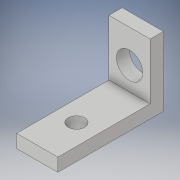
# Autodesk Inventor part: L形件
Saved by Autodesk Inventor 2017 (Build 210142000, 142)
## iProperties
Part Number: L形件
Material: 一般
Document SubType Name: Modeling
Designer: user
Density: 1 g/cm^3
Appearance: 預設
Author: user
Autodesk Inventor part; units mm, degrees
ref_plane "YZ Plane" through (0, 0, 0) normal (1, 0, 0) x (0, 1, 0)
ref_plane "XZ Plane" through (0, 0, 0) normal (0, 1, 0) x (-1, 0, 0)
ref_plane "XY Plane" through (0, 0, 0) normal (0, 0, 1) x (1, 0, 0)
sketch "草圖1" plane through (0, 0, 0) normal (1, 0, 0) x (0, 1, 0)
  line L0 (0, 0) -> (0, 32)
  line L1 (0, 32) -> (4, 32)
  line L2 (4, 32) -> (4, 4)
  line L3 (4, 4) -> (21, 4)
  line L4 (21, 4) -> (21, 0)
  line L5 (21, 0) -> (0, 0)
  dimension "d0" = 32
  dimension "d1" = 21
  dimension "d2" = 4
  dimension "d3" = 4
  constraints: 12 end point, 5 perpendicular, 1 vertical
  measures "d0" distance of L0.start L0.end
  measures "d1" distance of L4.end L0.start
  measures "d2" distance of L0.end L1.end
  measures "d3" distance between parallel lines of L5 L3
extrude "擠出1" add sketch "草圖1" along normal blind 12.5
sketch "草圖2" plane through (0, 4, 32) normal (0, 1, 0) x (1, 0, 0)
  circle A0 centre (6.25, 11.88) radius 2.5
  line L0 (0, 0) -> (12.5, 0) projected
  point P0 (0, 32)
  dimension "d6" = 5
  dimension "d7" = 11.88
  constraints: 1 centre point
  measures "d6" diameter of A0
  measures "d7" distance from line of A0.centre L0
extrude "擠出2" cut sketch "草圖2" against normal blind 12.5
sketch "草圖3" plane through (0, 4, 4) normal (0, 0, 1) x (1, 0, 0)
  circle A0 centre (6.25, 7) radius 4
  line L0 (0, 0) -> (0, 17) projected
  line L1 (0, -4) -> (12.5, -4) projected
  dimension "d10" = 8
  dimension "d11" = 6.25
  dimension "d12" = 11
  constraints: 1 centre point
  measures "d10" diameter of A0
  measures "d11" distance from line of L0 A0.centre
  measures "d12" distance from line of A0.centre L1
extrude "擠出3" cut sketch "草圖3" against normal blind 12.5
